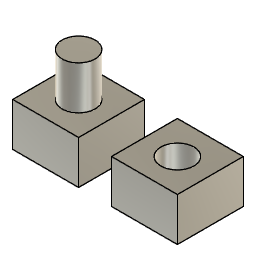
parametric_design_1 (Autodesk Fusion 360 design; units mm, degrees)
part number: 2025-09-03-23-28-59-638
Autodesk Fusion 360 part; units mm, degrees
sketch "Sketch1" plane through (0, 0, 0) normal (0, 0, 1) x (1, 0, 0)
  line L0 (17.5, -17.5) -> (-17.5, -17.5)
  line L1 (-17.5, -17.5) -> (-17.5, 17.5)
  line L2 (-17.5, 17.5) -> (17.5, 17.5)
  line L3 (17.5, 17.5) -> (17.5, -17.5)
  line L4 (17.5, -17.5) -> (-17.5, 17.5) construction
  line L5 (-17.5, -17.5) -> (17.5, 17.5) construction
  circle A0 centre (0, 0) radius 8.75
  line L6 (0, 0) -> (52.5, 0)
  line L7 (70, -17.5) -> (35, -17.5)
  line L8 (35, -17.5) -> (35, 17.5)
  line L9 (35, 17.5) -> (70, 17.5)
  line L10 (70, 17.5) -> (70, -17.5)
  line L11 (70, -17.5) -> (35, 17.5) construction
  line L12 (35, -17.5) -> (70, 17.5) construction
  circle A1 centre (52.5, 0) radius 8.75
  point P0 (52.5, 0)
  dimension "d6" = 35
  dimension "d7" = 35
  dimension "d8" = 17.5
  dimension "d13" = 52.5
  dimension "d14" = 35
  dimension "d15" = 35
  dimension "d16" = 17.5
  constraint horizontal L0
  constraint perpendicular L0 L1
  constraint parallel L0 L2
  constraint parallel L1 L3
  constraint coincident L4 A0.centre
  constraint coincident L5 A0.centre
  constraint coincident A0.centre L6.start
  constraint perpendicular L3 L6
  constraint horizontal L7
  constraint perpendicular L7 L8
  constraint parallel L7 L9
  constraint parallel L8 L10
  constraint coincident L11 P0
  constraint coincident L12 P0
  constraint coincident P0 L6.end
  measures "d6" distance of L1.end L2.end
  measures "d7" distance of L0.end L1.end
  measures "d8" diameter of A0
  measures "d13" distance of A0.centre P0
  measures "d14" distance of L8.end L9.end
  measures "d15" distance of L7.end L8.end
  measures "d16" diameter of A1
extrude "Extrude1" add sketch "Sketch1" along normal blind 23 contours L0 L1 L2 L3 makes body 1
extrude "Extrude2" add sketch "Sketch1" along normal blind 46 contours A0 bodies 1
extrude "Extrude4" add sketch "Sketch1" along normal blind 23 separate body contours L7 L8 L9 L10 makes body 2
equation "boxedge = 35 mm"
equation "boxlength = 23 mm"
equation "peg = boxlength * 2"
equation "distance = boxedge * 1.5"
equation "radius = boxedge / 2"
equation "d6 = boxedge"
equation "d7 = boxedge"
equation "d8 = radius"
equation "d9 = boxlength"
equation "d11 = peg"
equation "d13 = distance"
equation "d14 = boxedge"
equation "d15 = boxedge"
equation "d16 = radius"
equation "d19 = boxlength"
